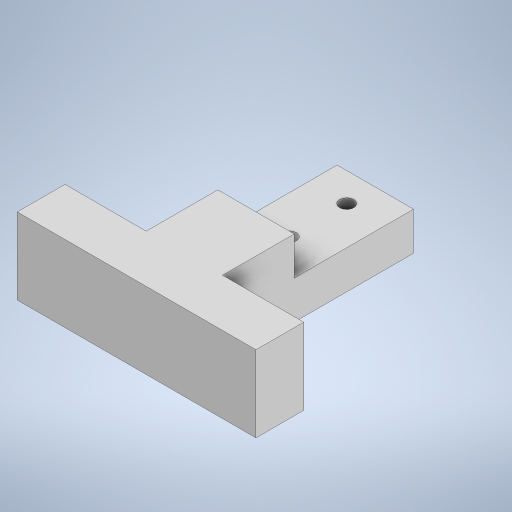
# Autodesk Inventor part: B1_head_T
Saved by Autodesk Inventor 2023.1 (Build 271208000, 208)
## iProperties
Created: 2023-06-14
Part Number: B1_head_T
Material: Generic
Document SubType Name: Modeling
Designer: zavrel
Density: 1 g/cm^3
Appearance: Default
Author: zavrel
Autodesk Inventor part; units mm, degrees
ref_plane "YZ Plane" through (0, 0, 0) normal (1, 0, 0) x (0, 1, 0)
ref_plane "XZ Plane" through (0, 0, 0) normal (0, 1, 0) x (-1, 0, 0)
ref_plane "XY Plane" through (0, 0, 0) normal (0, 0, 1) x (1, 0, 0)
sketch "Sketch1" plane through (0, 0, 0) normal (0, 1, 0) x (-1, 0, 0)
  line L0 (0, -50) -> (8, -50)
  line L1 (8, -50) -> (8, -10)
  line L2 (8, -10) -> (25, -10)
  line L3 (25, -10) -> (25, 0)
  line L4 (25, 0) -> (0, 0)
  line L5 (0, 0) -> (0, -50) construction
  line L6 (0, -50) -> (-8, -50)
  line L7 (-8, -50) -> (-8, -10)
  line L8 (-8, -10) -> (-25, -10)
  line L9 (-25, -10) -> (-25, 0)
  line L10 (-25, 0) -> (0, 0)
  point P0 (0, 0)
  point P1 (4, -50)
  point P2 (16.5, -10)
  point P3 (25, -5)
  point P4 (-25, -5)
  dimension "d0" = 16
  dimension "d1" = 50
  dimension "d2" = 10
  dimension "d3" = 50
  constraints: 22 end point, 4 midpoint, 4 perpendicular, 4 symmetric about line, 1 coincident, 1 horizontal, 1 vertical
  measures "d0" distance between parallel lines of L7 L1
  measures "d1" distance from line of L10 point (4, -50)
  measures "d2" distance from line of point (16.5, -10) L4
  measures "d3" distance of point (25, -5) point (-25, -5)
extrude "Extrusion1" add sketch "Sketch1" along normal blind 16
sketch "Sketch2" plane through (0, 16, 0) normal (0, 1, 0) x (1, 0, 0)
  line L0 (8, 50) -> (-8, 50) projected
  line L1 (-8, 50) -> (-8, 10) projected
  line L2 (-8, 10) -> (-25, 10) projected
  line L3 (-25, 10) -> (-25, 0) projected
  line L4 (-25, 0) -> (25, 0) projected
  line L5 (25, 0) -> (25, 10) projected
  line L6 (25, 10) -> (8, 10) projected
  line L7 (8, 10) -> (8, 50) projected
  line L8 (8, 10) -> (8, 50) projected
  line L9 (-8, 50) -> (8, 50)
  line L10 (8, 50) -> (8, 25)
  line L11 (8, 25) -> (-8, 25)
  line L12 (-8, 25) -> (-8, 50)
  point P0 (0, 0)
  dimension "d6" = 25
  constraints: 8 end point, 2 parallel, 1 horizontal, 1 perpendicular, 1 point on line
  measures "d6" distance between parallel lines of L0 L11
extrude "Extrusion2" cut sketch "Sketch2" against normal blind 8 contours L7 L11 L1 L0
sketch "Sketch3" plane through (0, 0, 0) normal (0, -1, 0) x (1, 0, 0)
  line L0 (8, -50) -> (-8, -50) projected
  line L1 (8, -10) -> (8, -50) projected
  line L2 (25, -10) -> (8, -10) projected
  line L3 (25, 0) -> (25, -10) projected
  line L4 (-25, 0) -> (25, 0) projected
  line L5 (-25, -10) -> (-25, 0) projected
  line L6 (-8, -10) -> (-25, -10) projected
  line L7 (-8, -50) -> (-8, -10) projected
  circle A0 centre (0, -44) radius 1.5
  circle A1 centre (0, -32) radius 1.5
  point P0 (0, 0)
  dimension "d9" = 3
  dimension "d10" = 6
  dimension "d11" = 12
  constraints: 2 centre point, 1 equal radius
  measures "d9" diameter of A0
  measures "d10" distance from line of A0.centre L0
  measures "d11" distance of A0.centre A1.centre
extrude "Extrusion3" cut sketch "Sketch3" against normal through all contours A0 | A1
sketch "Sketch4" plane through (0, 0, 0) normal (0, -1, 0) x (1, 0, 0)
  circle A0 centre (0, -32) radius 1.5 projected
  circle A1 centre (0, -44) radius 1.5 projected
  line L0 (8, -50) -> (-8, -50) projected
  line L1 (8, -10) -> (8, -50) projected
  line L2 (25, -10) -> (8, -10) projected
  line L3 (25, 0) -> (25, -10) projected
  line L4 (-25, 0) -> (25, 0) projected
  line L5 (-25, -10) -> (-25, 0) projected
  line L6 (-8, -10) -> (-25, -10) projected
  line L7 (-8, -50) -> (-8, -10) projected
  circle A2 centre (0, -44) radius 3
  circle A3 centre (0, -32) radius 1.5 projected
  circle A4 centre (0, -32) radius 3
  point P0 (0, 0)
  dimension "d14" = 6
  constraints: 2 centre point, 2 coincident, 1 equal radius
  measures "d14" diameter of A4
extrude "Extrusion4" cut sketch "Sketch4" against normal blind 3 contours A2 | A4
body "Solid1"
